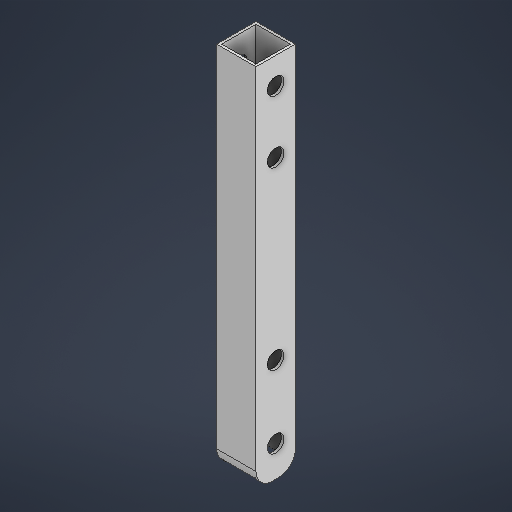
# Autodesk Inventor part: Pedalbox_V2_Brake_Extrusion
Saved by Autodesk Inventor 2026.1 (Build 301233000, 233)
## iProperties
Created: 2026-09-15
Part Number: Pedalbox_V2_Brake_Extrusion
Material: Generic
Document SubType Name: Modeling
Designer: share
Density: 1 g/cm^3
Appearance: Default
Author: share
Autodesk Inventor part; units mm, degrees
ref_plane "YZ Plane" through (0, 0, 0) normal (1, 0, 0) x (0, 1, 0)
ref_plane "XZ Plane" through (0, 0, 0) normal (0, 1, 0) x (-1, 0, 0)
ref_plane "XY Plane" through (0, 0, 0) normal (0, 0, 1) x (1, 0, 0)
sketch "Sketch4" plane through (0, 0, 0) normal (0, 1, 0) x (-1, 0, 0)
  line L0 (-9.525, -9.525) -> (9.525, -9.525)
  line L1 (9.525, -9.525) -> (9.525, 9.525)
  line L2 (9.525, 9.525) -> (-9.525, 9.525)
  line L3 (-9.525, 9.525) -> (-9.525, -9.525)
  line L4 (0, -13.335) -> (0, 13.335) construction
  line L5 (13.335, 0) -> (-13.335, 0) construction
  line L6 (-8.3058, 8.3058) -> (8.3058, 8.3058)
  line L7 (8.3058, 8.3058) -> (8.3058, -8.3058)
  line L8 (8.3058, -8.3058) -> (-8.3058, -8.3058)
  line L9 (-8.3058, -8.3058) -> (-8.3058, 8.3058)
  point P0 (0, 0)
  dimension "d44" = 19.05
  dimension "d45" = 1.2192
  constraints: 16 end point, 4 parallel, 3 perpendicular, 1 horizontal, 5 other
  measures "d44" distance between parallel lines of L3 L1
  measures "d45" distance between parallel lines of L6 L2
extrude "Extrusion2" add sketch "Sketch4" along normal blind 177.8
sketch "Sketch5" plane through (0, 0, 0) normal (1, 0, 0) x (0, 1, 0)
  line L0 (0, 115.5) -> (0, -115.5) construction
  line L1 (-33, 0) -> (198, 0) construction
  line L2 (165, 0) -> (135, 0)
  point P0 (0, 0)
  point P1 (50, 0)
  point P2 (15, 0)
  point P3 (150, 0)
  dimension "d48" = 15
  dimension "d49" = 50
  dimension "d50" = 30
  dimension "d51" = 135
  dimension "d59" = 150
  constraints: 4 point on line, 2 end point, 1 horizontal, 1 midpoint
  measures "d48" distance from line of L0 point (15, 0)
  measures "d49" distance from line of L0 point (50, 0)
  measures "d50" distance of L2.end L2.start
  measures "d51" distance from line of L0 L2.end
  measures "d59" distance from line of point (150, 0) L0
hole "Hole2" at (0, 50, 0) at (0, 15, 0) at (0, 165, 0) at (0, 135, 0) direction (-1, 0, 0) diameter 8 end through all both
fillet "Fillet2" radius 8 2 edges at (0, 0, -9.525) (0, 0, 9.525)
body "Solid2"
